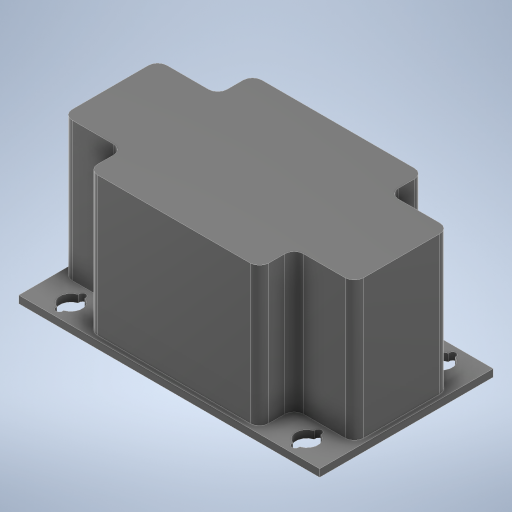
# Autodesk Inventor part: SUSTAINA-POWER-LOGGING-BOARD
Saved by Autodesk Inventor 2024.2 (Build 282272000, 272)
## iProperties
Created: 2024-01-24
Part Number: SUSTAINA-POWER-LOGGING-BOARD
Material: Acetal Resin, Black
Document SubType Name: Modeling
Designer: Masato Kubotera
Appearance: Smooth - Black
Surface Area: 123.153 cm^2
Volume: 52.2328 cm^3
Author: Masato Kubotera
Autodesk Inventor part; units mm, degrees
ref_plane "YZ Plane" through (0, 0, 0) normal (1, 0, 0) x (0, 1, 0)
ref_plane "XZ Plane" through (0, 0, 0) normal (0, 1, 0) x (-1, 0, 0)
ref_plane "XY Plane" through (0, 0, 0) normal (0, 0, 1) x (1, 0, 0)
sketch "Sketch1" plane through (0, 0, 0) normal (0, 0, 1) x (1, 0, 0)
  line L0 (18.75, 32.5) -> (-18.75, 32.5)
  line L1 (-18.75, 32.5) -> (-18.75, -32.5)
  line L2 (-18.75, -32.5) -> (18.75, -32.5)
  line L3 (18.75, -32.5) -> (18.75, 32.5)
  line L4 (18.75, 32.5) -> (-18.75, -32.5) construction
  line L5 (-18.75, 32.5) -> (18.75, -32.5) construction
  line L6 (-14.5, 25.5) -> (14.5, 25.5) construction
  line L7 (14.5, 25.5) -> (14.5, -25.5) construction
  line L8 (14.5, -25.5) -> (-14.5, -25.5) construction
  line L9 (-14.5, -25.5) -> (-14.5, 25.5) construction
  line L10 (-14.5, 25.5) -> (14.5, -25.5) construction
  line L11 (14.5, 25.5) -> (-14.5, -25.5) construction
  line L12 (18.75, 0) -> (-18.75, 0) construction
  line L13 (0, 32.5) -> (0, -32.5) construction
  circle A0 centre (14.5, 25.5) radius 2.4
  circle A1 centre (-14.5, 25.5) radius 2.4
  circle A2 centre (14.5, -25.5) radius 2.4
  circle A3 centre (-14.5, -25.5) radius 2.4
  line L14 (14.5, 31.5) -> (14.5, 19.5) construction
  line L15 (17.75, 18.5) -> (-17.75, 18.5)
  line L16 (-17.75, 18.5) -> (-17.75, -18.5)
  line L17 (-17.75, -18.5) -> (17.75, -18.5)
  line L18 (17.75, -18.5) -> (17.75, 18.5)
  line L19 (17.75, 18.5) -> (-17.75, -18.5) construction
  line L20 (-17.75, 18.5) -> (17.75, -18.5) construction
  line L21 (10.25, 18.5) -> (10.25, 31.5)
  line L22 (10.25, 31.5) -> (-10.25, 31.5)
  line L23 (-10.25, 31.5) -> (-10.25, 18.5)
  line L24 (10.25, -18.5) -> (10.25, -31.5)
  line L25 (10.25, -31.5) -> (-10.25, -31.5)
  line L26 (-10.25, -31.5) -> (-10.25, -18.5)
  arc A4 (12.2105, 26.2199) -> (12.2105, 24.7801) centre (12, 25.5) ccw
  arc A5 (16.7895, 24.7801) -> (16.7895, 26.2199) centre (17, 25.5) ccw
  arc A6 (12.2105, -24.7801) -> (12.2105, -26.2199) centre (12, -25.5) ccw
  arc A7 (16.7895, -26.2199) -> (16.7895, -24.7801) centre (17, -25.5) ccw
  arc A8 (-12.2105, 24.7801) -> (-12.2105, 26.2199) centre (-12, 25.5) ccw
  arc A9 (-16.7895, 26.2199) -> (-16.7895, 24.7801) centre (-17, 25.5) ccw
  arc A10 (-12.2105, -26.2199) -> (-12.2105, -24.7801) centre (-12, -25.5) ccw
  arc A11 (-16.7895, -24.7801) -> (-16.7895, -26.2199) centre (-17, -25.5) ccw
  point P0 (0, 0)
  point P1 (10.25, -18.5)
  point P2 (17.75, 25.5)
  point P3 (11.25, 25.5)
  point P4 (16.7895, 26.2199)
  point P5 (16.7895, 24.7801)
  point P6 (16.7895, -24.7801)
  point P7 (16.7895, -26.2199)
  point P8 (12.2105, -26.2199)
  point P9 (12.2105, -24.7801)
  point P10 (-16.7895, -26.2199)
  point P11 (-16.7895, -24.7801)
  point P12 (-12.2105, -24.7801)
  point P13 (-12.2105, -26.2199)
  point P14 (-16.7895, 24.7801)
  point P15 (-16.7895, 26.2199)
  point P16 (-12.2105, 26.2199)
  point P17 (-12.2105, 24.7801)
  dimension "d0" = 37.5
  dimension "d1" = 65
  dimension "d19" = 4.8
  dimension "d33" = 51
  dimension "d34" = 29
  dimension "d38" = 1
  dimension "d43" = 1
  dimension "d44" = 1
  dimension "d46" = 6.5
  dimension "d47" = 1.5
  dimension "d48" = 1
  dimension "d50" = 14
  constraints: 54 end point, 28 symmetric about line, 20 point on circle, 12 centre point, 11 midpoint, 6 coincident, 6 parallel, 4 horizontal, 3 perpendicular, 3 point on line, 3 vertical, 13 other
  measures "d0" distance of L2.end L1.end
  measures "d1" distance of L1.end L0.end
  measures "d19" diameter of A0
  measures "d33" distance of L8.end L6.start
  measures "d34" distance of L7.end L8.end
  measures "d38" distance between parallel lines of L3 L18
  measures "d43" distance from line of L0 L14.start
  measures "d44" distance between parallel lines of L0 L22
  measures "d46" distance of point (17.75, 25.5) point (11.25, 25.5)
  measures "d47" diameter of A4
  measures "d48" distance from line of L3 point (17.75, 25.5)
  measures "d50" diameter of L0 L6
extrude "Extrusion1" add sketch "Sketch1" along normal blind 1.6 contours L3 L2 L1 L0 | L18 L17 L16 L15 | L15 L23 L22 L21 | L24 L25 L26 L17
extrude "Extrusion2" add sketch "Sketch1" along normal blind 31.6 contours L18 L17 L16 L15 | L15 L23 L22 L21 | L24 L25 L26 L17
fillet "Fillet1" radius 2 12 edges at (17.75, -18.5, 16.6) (17.75, 18.5, 16.6) (-17.75, -18.5, 16.6) (-17.75, 18.5, 16.6) (10.25, 18.5, 16.6) (10.25, -18.5, 16.6) (10.25, -31.5, 16.6) (-10.25, -31.5, 16.6) (-10.25, -18.5, 16.6) (-10.25, 18.5, 16.6) (-10.25, 31.5, 16.6) (10.25, 31.5, 16.6)
body "Solid1"
